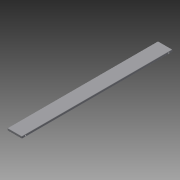
# Autodesk Inventor part: CeramicModelv2
Saved by Autodesk Inventor 2015 SP1 (Build 190203100, 203)
## iProperties
Created: 2015-11-12
Part Number: CeramicModelv2
Material: Generic
Document SubType Name: Modeling
Designer: I Rabey
Density: 1 g/cm^3
Appearance: Default
Author: I Rabey
Autodesk Inventor part; units mm, degrees
ref_plane "YZ Plane" through (0, 0, 0) normal (1, 0, 0) x (0, 1, 0)
ref_plane "XZ Plane" through (0, 0, 0) normal (0, 1, 0) x (-1, 0, 0)
ref_plane "XY Plane" through (0, 0, 0) normal (0, 0, 1) x (1, 0, 0)
sketch "Sketch1" plane through (0, 0, 0) normal (0, 1, 0) x (-1, 0, 0)
  line L0 (-40, 417.5) -> (40, 417.5)
  line L1 (40, 417.5) -> (40, -417.5)
  line L2 (40, -417.5) -> (-40, -417.5)
  line L3 (-40, -417.5) -> (-40, 417.5)
  line L4 (-40, 417.5) -> (40, -417.5) construction
  line L5 (40, 417.5) -> (-40, -417.5) construction
  point P0 (0, 0)
  dimension "d0" = 80
  dimension "d1" = 835
  constraints: 12 end point, 2 midpoint, 2 parallel, 1 horizontal, 1 perpendicular
  measures "d0" distance of L1.end L2.end
  measures "d1" distance of L0.end L1.end
extrude "Extrusion1" add sketch "Sketch1" along normal blind 12
fillet "Fillet1" radius 2 1 edges at (40, 6, 417.5)
fillet "Fillet2" radius 2 3 edges at (39.4142, 12, 416.9142) (-1, 12, 417.5) (40, 12, -1)
fillet "Fillet3" radius 2 3 edges at (39.4142, 0, 416.9142) (-1, 0, 417.5) (40, 0, -1)
fillet "Fillet4" radius 2 5 edges at (-40, 6, 417.5) (-40, 0.5858, 416.9142) (-40, 0, -1) (-40, 12, -1) (-40, 11.4142, 416.9142)
fillet "Fillet5" radius 2 8 edges at (-39.4142, 11.4142, -417.5) (0, 12, -417.5) (39.4142, 11.4142, -417.5) (40, 6, -417.5) (39.4142, 0.5858, -417.5) (0, 0, -417.5) (-39.4142, 0.5858, -417.5) (-40, 6, -417.5)
sketch "Sketch2" plane through (-40, 2, -415.5) normal (-1, 0, 0) x (0, 0, 1)
  circle A0 centre (18, 4) radius 4
  line L0 (-2, 8) -> (-2, 0) projected
  line L1 (0, -2) -> (831, -2) projected
  circle A1 centre (813, 4) radius 4
  line L2 (833, 0) -> (833, 8) projected
  line L3 (831, 10) -> (0, 10) projected
  point P0 (415.5, -2)
  dimension "d9" = 8
  dimension "d10" = 20
  dimension "d11" = 6
  dimension "d12" = 8
  dimension "d13" = 20
  dimension "d21" = 6
  constraints: 2 centre point
  measures "d9" diameter of A0
  measures "d10" distance from line of L0 A0.centre
  measures "d11" distance from line of L1 A0.centre
  measures "d12" diameter of A1
  measures "d13" distance from line of L2 A1.centre
  measures "d21" distance from line of L3 A1.centre
hole "Hole1" at (-40, 6, -397.5) at (-40, 6, 397.5) direction (1, 0, 0) diameter 8 end through all
equation "\"d12\" = d9"
equation "\"d13\" = d10"
equation "\"d21\" = d11"
body "Solid1"
